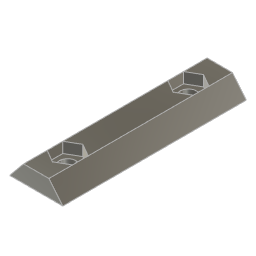
rail nut m3 (Autodesk Fusion 360 design; units mm, degrees)
Autodesk Fusion 360 part; units mm, degrees
sketch "Sketch1" plane through (0, 0, 0) normal (0, 1, 0) x (1, 0, 0)
  line L0 (0, 0) -> (5.5, 0)
  line L1 (0, -3.5) -> (2.625, -3.5)
  line L2 (2.625, -3.5) -> (5.5, 0)
  line L3 (0, -1.75) -> (0, -22.5)
  line L4 (0, -3.5) -> (-2.625, -3.5)
  line L5 (-2.625, -3.5) -> (-5.5, 0)
  line L6 (0, 0) -> (-5.5, 0)
  dimension "d1" = 5.5
  dimension "d2" = 2.625
  dimension "d3" = 3.5
  constraint coincident L0.start L6.start
  constraint horizontal L0
  constraint parallel L0 L1
  constraint symmetric L0.start L3 L6.start
  constraint symmetric L0.end L3 L5.end
  constraint symmetric L1.start L3 L4.start
  constraint symmetric L1.end L3 L4.end
  measures "d1" distance of L0.start L0.end
  measures "d2" distance of L1.start L1.end
  measures "d3" distance of L0 L1
extrude "Extrude1" add sketch "Sketch1" along normal blind 38
sketch "Sketch2" plane through (0, 0, 3.5) normal (0, 0, 1) x (-1, 0, 0)
  line L0 (2.625, 0) -> (-2.625, 0)
  line L1 (-2.625, 0) -> (-2.625, -38)
  line L2 (-2.625, -38) -> (2.625, -38)
  line L3 (2.625, -38) -> (2.625, 0)
  line L4 (0, -38) -> (0, 0) construction
  line L5 (2.72, -29.9296) -> (0, -28.3592)
  line L6 (0, -28.3592) -> (-2.72, -29.9296)
  line L7 (-2.72, -29.9296) -> (-2.72, -33.0704)
  line L8 (-2.72, -33.0704) -> (0, -34.6408)
  line L9 (0, -34.6408) -> (2.72, -33.0704)
  line L10 (2.72, -33.0704) -> (2.72, -29.9296)
  line L11 (2.72, -4.9296) -> (0, -3.3592)
  line L12 (0, -3.3592) -> (-2.72, -4.9296)
  line L13 (-2.72, -4.9296) -> (-2.72, -8.0704)
  line L14 (-2.72, -8.0704) -> (0, -9.6408)
  line L15 (0, -9.6408) -> (2.72, -8.0704)
  line L16 (2.72, -8.0704) -> (2.72, -4.9296)
  point P0 (0, -31.5)
  point P1 (0, -6.5)
  dimension "d6" = 2.72
  dimension "d7" = 2.72
  dimension "d8" = 25
  dimension "d9" = 6.5
  constraint midpoint L2 L4.start
  constraint coincident L4.end origin
  constraint coincident L4 P0
  constraint coincident L4 P1
  constraint vertical L10
  constraint vertical L16
  measures "d6" distance of P0 L10
  measures "d7" distance of P1 L16
  measures "d8" distance of P0 P1
  measures "d9" distance of L2 P0
extrude "Extrude2" cut sketch "Sketch2" against normal blind 2.2 contours L1 L3 L11 L12 L14 L15 | L1 L3 L5 L6 L8 L9
hole "Hole1" at (0, 31.5, 3.5) at (0, 6.5, 3.5) direction (0, 0, -1) diameter 3.4 depth 16 tip angle 118
equation "d2 = ( 5.25 / 2 ) * 1 mm"
equation "d6 = ( 5.44 / 2 ) * 1 mm"
equation "d7 = ( 5.44 / 2 ) * 1 mm"
